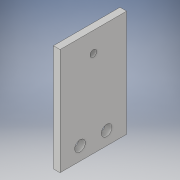
# Autodesk Inventor part: Stuetzplatte
Saved by Autodesk Inventor 2018 (Build 220112000, 112)
## iProperties
Created: 2018-01-30
Part Number: Stuetzplatte
Material: Generisch
Document SubType Name: Modeling
Designer: Julian
Density: 1 g/cm^3
Appearance: Vorgabe
Author: Julian
Autodesk Inventor part; units mm, degrees
ref_plane "YZ Plane" through (0, 0, 0) normal (1, 0, 0) x (0, 1, 0)
ref_plane "XZ Plane" through (0, 0, 0) normal (0, 1, 0) x (-1, 0, 0)
ref_plane "XY Plane" through (0, 0, 0) normal (0, 0, 1) x (1, 0, 0)
sketch "Skizze1" plane through (0, 0, 0) normal (1, 0, 0) x (0, 1, 0)
  line L0 (0, 0) -> (50, 0)
  line L1 (50, 0) -> (50, -80)
  line L2 (50, -80) -> (0, -80)
  line L3 (0, -80) -> (0, 0)
  dimension "d0" = 50
  dimension "d1" = 80
  constraints: 8 end point, 2 parallel, 1 horizontal, 1 perpendicular
  measures "d0" distance of L1.end L2.end
  measures "d1" distance of L0.end L1.end
extrude "Extrusion1" add sketch "Skizze1" along normal blind 5
sketch "Skizze2" plane through (5, 0, 0) normal (1, 0, 0) x (0, 0, -1)
  line L0 (0, 0) -> (80, 0) projected
  line L1 (80, 0) -> (70, 0)
  line L2 (70, 0) -> (70, 15)
  line L3 (70, 15) -> (70, 35)
  line L4 (70, 35) -> (70, 50)
  dimension "d4" = 10
  dimension "d5" = 15
  dimension "d6" = 20
  dimension "d7" = 15
  constraints: 8 end point, 3 point on line, 1 perpendicular
  measures "d4" distance of L0.end L1.end
  measures "d5" distance of L1.end L2.end
  measures "d6" distance of L2.end L3.end
  measures "d7" distance of L3.end L4.end
hole "Bohrung1" at (5, 35, -70) at (5, 15, -70) direction (-1, 0, 0) diameter 8 depth 8 tip angle 118
sketch "Skizze3" plane through (5, 0, 0) normal (1, 0, 0) x (0, 0, -1)
  line L0 (0, 0) -> (0, 25)
  line L1 (0, 50) -> (0, 0) projected
  line L2 (0, 25) -> (15, 25)
  circle A0 centre (15, 25) radius 2.5
  dimension "d15" = 25
  dimension "d16" = 15
  dimension "d17" = 5
  constraints: 4 end point, 1 centre point, 1 coincident, 1 midpoint, 1 perpendicular
  measures "d15" distance of L0.start L0.end
  measures "d16" distance of L0.end L2.end
  measures "d17" diameter of A0
extrude "Extrusion2" cut sketch "Skizze3" against normal blind 10
